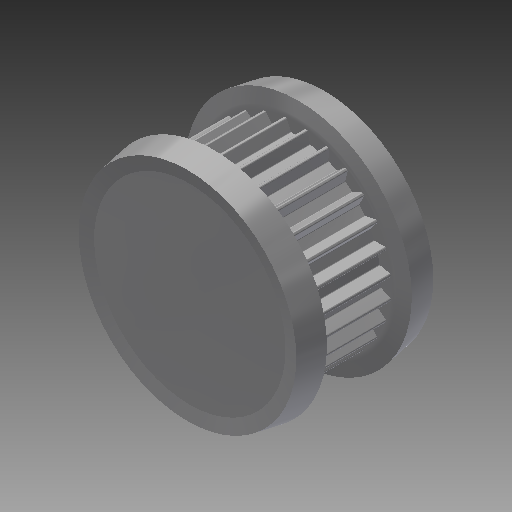
# Autodesk Inventor part: Synchronous Pulley1
Saved by Autodesk Inventor 2017 SP1 (Build 210196100, 196)
## iProperties
Created: 2017-11-17
Part Number: Synchronous Pulley1
Material: Steel
Document SubType Name: Modeling
Designer: Biscuit
Density: 1 g/cm^3
Appearance: Steel
CustomPartVersion: 1
Author: Biscuit
Autodesk Inventor part; units mm, degrees
ref_plane "YZ Plane" through (0, 0, 0) normal (1, 0, 0) x (0, 1, 0)
ref_plane "XZ Plane" through (0, 0, 0) normal (0, 1, 0) x (-1, 0, 0)
ref_plane "XY Plane" through (0, 0, 0) normal (0, 0, 1) x (1, 0, 0)
sketch "Pulley Sketch" plane through (0, 0, 0) normal (0, 0, 1) x (1, 0, 0)
  circle A0 centre (0, 0) radius 11.1408 construction
  circle A1 centre (0, 0) radius 10.8408
  circle A2 centre (0, 0) radius 9.6408
  line L0 (-1.0603, 10.7889) -> (-0.525, 9.6408)
  line L1 (-0.525, 9.6408) -> (0.525, 9.6408)
  line L2 (0.525, 9.6408) -> (1.0603, 10.7889)
  line L3 (0, 0) -> (0, 10.8408) construction
  point P0 (0, 9.6408)
  dimension "d0" = 22.2817
  dimension "d1" = 0.3
  dimension "d2" = 1.2
  dimension "d3" = 50
  dimension "d4" = 1.05
  constraints: 8 end point, 3 coincident, 3 point on circle, 2 centre point, 1 horizontal, 1 midpoint, 1 point on line, 1 vertical, 1 vertical alignment, 3 other
  measures "d0" diameter of A0
  measures "d1" radial gap between concentric circles of A0 A1
  measures "d3" angle of L2 L0
  measures "d4" distance of L0.end L1.end
extrude "Base Body" add sketch "Pulley Sketch" along normal mid plane 9 contours A2 | A1 L0 L1 L2 | L2 L1 L0 A1
extrude "Tooth" cut sketch "Pulley Sketch" along normal through all both and the other way through all contours L2 L1 L0 A1 picked at (0, 10.4369)
fillet "Tooth Fillet" radius 0.1 2 edges at (0.525, 9.6408, 0) (-0.525, 9.6408, 0)
fillet "Tooth Fillet" radius 0.15 4 edges at (-1.0603, 10.7889, 2.25) (-1.0603, 10.7889, -2.25) (1.0603, 10.7889, 2.25) (1.0603, 10.7889, -2.25)
pattern_circular "Teeth" count 28 over 360 about axis through (0, 0, -10) along (0, 0, 1) of "Tooth", "Tooth Fillet"
pulley flange "Left flange" diameter 21.6817 height 2 thickness 3 bend angle 10 centre (0, 0, -4.5) toward (0, 0, -1)
pulley flange "Right flange" diameter 21.6817 height 2 thickness 3 bend angle 10 centre (0, 0, 4.5) toward (0, 0, 1)
equation "\"d1\" = da_a"
equation "\"d2\" = da_hg"
equation "\"d3\" = 2 * da_fi"
equation "\"d4\" = da_bw"
equation "\"d5\" = da_bf"
equation "\"d7\" = da_bf"
equation "\"d9\" = da_rb"
equation "\"d10\" = da_rt"
equation "\"da_pb\" = 2.5"
equation "\"da_fi\" = 25deg"
equation "\"da_hg\" = 1.2"
equation "\"da_bw\" = 1.05"
equation "\"da_rb\" = 0.1"
equation "\"da_rt\" = 0.15"
equation "\"da_a\" = 0.3"
equation "\"da_bf\" = 9"
equation "\"da_wf\" = 3"
equation "\"da_hf\" = 2"
body "Solid1"
